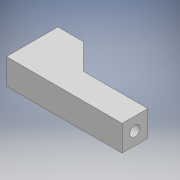
# Autodesk Inventor part: support 1
Saved by Autodesk Inventor 2017 (Build 210142000, 142)
## iProperties
Created: 2018-09-04
Part Number: support 1
Material: Generic
Document SubType Name: Modeling
Designer: jakub.tomczynski
Density: 1 g/cm^3
Appearance: Default
Author: jakub.tomczynski
## iProperties of the stored document support 1_3DPrint.ipt
Created: 2018-09-04
Part Number: support 1_3DPrint
Material: Generic
Document SubType Name: Modeling
Designer: jakub.tomczynski
Density: 1 g/cm^3
Appearance: Default
Author: jakub.tomczynski
Autodesk Inventor part; units mm, degrees
ref_plane "YZ Plane" through (0, 0, 0) normal (1, 0, 0) x (0, 1, 0)
ref_plane "XZ Plane" through (0, 0, 0) normal (0, 1, 0) x (-1, 0, 0)
ref_plane "XY Plane" through (0, 0, 0) normal (0, 0, 1) x (1, 0, 0)
sketch "Sketch1" plane through (0, 0, 0) normal (0, 0, 1) x (1, 0, 0)
  line L0 (0, 0) -> (0, 8)
  line L1 (0, 8) -> (4, 8)
  line L2 (4, 8) -> (8, 4)
  line L3 (8, 4) -> (18, 4)
  line L4 (18, 4) -> (18, 0)
  line L5 (18, 0) -> (0, 0)
  dimension "d0" = 18
  dimension "d1" = 4
  dimension "d2" = 8
  dimension "d3" = 4
  dimension "d4" = 45
  constraints: 12 end point, 3 perpendicular, 1 parallel, 1 vertical
  measures "d0" distance between parallel lines of L4 L0
  measures "d1" distance between parallel lines of L5 L3
  measures "d2" distance between parallel lines of L5 L1
  measures "d3" distance of L0.end L1.end
  measures "d4" angle of L1 L2
extrude "Extrusion1" add sketch "Sketch1" along normal blind 4
sketch "Sketch2" plane through (0, 0, 0) normal (-1, 0, 0) x (0, 0, 1)
  line L0 (0, 0) -> (0, 8) projected
  line L1 (0, 0) -> (4, 0) projected
  line L2 (4, 8) -> (4, 0) projected
  line L3 (0, 8) -> (4, 8) projected
  line L4 (2, 0) -> (2, 8) construction
  line L5 (0, 4) -> (4, 4) construction
  point P0 (2, 2)
  point P1 (2, 6)
  dimension "d7" = 4
  constraints: 4 end point, 4 midpoint, 2 point on line, 1 symmetric about line
  measures "d7" distance of point (2, 6) point (2, 2)
hole "Hole1" at (0, 2, 2) at (0, 6, 2) direction (1, 0, 0) diameter 1.6 depth 5 tip angle 118
sketch "Sketch3" plane through (18, 0, 0) normal (1, 0, 0) x (0, 0, -1)
  line L0 (0, 4) -> (0, 0) projected
  line L1 (0, 4) -> (-4, 4) projected
  line L2 (-4, 0) -> (-4, 4) projected
  line L3 (0, 0) -> (-4, 0) projected
  line L4 (0, 0) -> (-4, 4) construction
  point P0 (0, 0)
  point P1 (-2, 2)
  constraints: 2 end point, 1 midpoint
hole "Hole2" at (18, 2, 2) direction (-1, 0, 0) diameter 1.6 depth 5 tip angle 118
body "Solid1"
